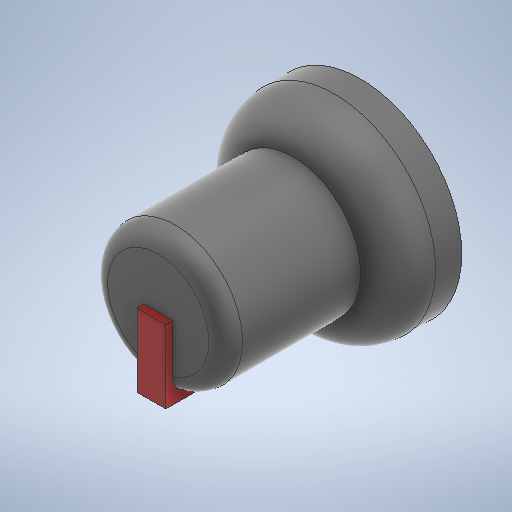
# Autodesk Inventor part: VOL KNOB
Saved by Autodesk Inventor 2025 (Build 290162000, 162)
## iProperties
Created: 2025-05-10
Part Number: VOL KNOB
Material: Generic
Document SubType Name: Modeling
Designer: thesn
Density: 1 g/cm^3
Appearance: Default
Author: thesn
Autodesk Inventor part; units mm, degrees
ref_plane "YZ Plane" through (0, 0, 0) normal (1, 0, 0) x (0, 1, 0)
ref_plane "XZ Plane" through (0, 0, 0) normal (0, 1, 0) x (-1, 0, 0)
ref_plane "XY Plane" through (0, 0, 0) normal (0, 0, 1) x (1, 0, 0)
sketch "Sketch1" plane through (0, 0, 0) normal (0, 0, 1) x (1, 0, 0)
  circle A0 centre (0, 0) radius 7.62
  circle A1 centre (0, 0) radius 5.08
  dimension "d0" = 15.24
  dimension "d1" = 10.16
  constraints: 2 centre point, 2 coincident
  measures "d0" diameter of A0
  measures "d1" diameter of A1
extrude "Extrusion1" add sketch "Sketch1" along normal blind 5.08 contours A0 | A1
extrude "Extrusion2" add sketch "Sketch1" along normal blind 15.24 contours A1
fillet "Fillet1" radius 3.175 1 edges at (-7.62, 0, 5.08)
fillet "Fillet2" radius 1.27 1 edges at (-5.08, 0, 15.24)
sketch "Sketch2" plane through (0, 0, 15.24) normal (0, 0, 1) x (1, 0, 0)
  line L0 (-1.0825, -0.0027) -> (1.0835, -0.0027)
  line L1 (1.0835, -0.0027) -> (1.0835, -5.4984)
  line L2 (1.0835, -5.4984) -> (-1.0825, -5.4984)
  line L3 (-1.0825, -5.4984) -> (-1.0825, -0.0027)
  point P0 (0, 0)
  point P1 (0.0005, -5.4984)
  point P2 (0.0005, -0.0027)
  dimension "d8" = 2.166
  dimension "d9" = 5.4958
  constraints: 8 end point, 2 midpoint, 2 parallel, 1 horizontal, 1 perpendicular
  measures "d8" distance between parallel lines of L1 L3
  measures "d9" distance of point (0, -5.498) point (0, -0.003)
extrude "Extrusion3" add sketch "Sketch2" along normal blind 0.508 and the other way blind 12.7
sketch "Sketch3" plane through (0, 0, 0) normal (0, 0, -1) x (-1, 0, 0)
  line L0 (-6.251, 1.1807) -> (3.3004, 1.1807) construction
  line L1 (3.3004, 1.1807) -> (3.3004, -0.1036) construction
  line L2 (3.3004, -0.1036) -> (-6.251, -0.1036) construction
  line L3 (-6.251, -0.1036) -> (-6.251, 1.1807) construction
  line L4 (-6.2543, 0.6467) -> (-6.083, 1.1547)
  line L5 (-6.083, 1.1547) -> (-5.9999, 1.1547)
  line L6 (-5.9999, 1.1547) -> (-5.8286, 0.6467)
  line L7 (-5.8286, 0.6467) -> (-5.8998, 0.6467)
  line L8 (-5.8998, 0.6467) -> (-5.9459, 0.7888)
  line L9 (-5.9459, 0.7888) -> (-6.1398, 0.7888)
  line L10 (-6.1398, 0.7888) -> (-6.1859, 0.6467)
  line L11 (-6.1859, 0.6467) -> (-6.2543, 0.6467)
  line L12 (-5.9645, 0.8464) -> (-6.0431, 1.0856)
  line L13 (-6.0431, 1.0856) -> (-6.1213, 0.8464)
  line L14 (-6.1213, 0.8464) -> (-5.9645, 0.8464)
  line L15 (-5.4923, 0.6467) -> (-5.5565, 0.6467)
  line L16 (-5.5565, 0.6467) -> (-5.5565, 0.6854)
  spline S0 degree 2 poles (-5.5565, 0.6854) (-5.5713, 0.6731) (-5.5931, 0.6566) (-5.608, 0.6496) knots 0 0 0 1 2 2 2
  spline S1 degree 2 poles (-5.608, 0.6496) (-5.6216, 0.643) (-5.6508, 0.636) (-5.6701, 0.636) knots 0 0 0 1 2 2 2
  spline S2 degree 2 poles (-5.6701, 0.636) (-5.7014, 0.636) (-5.7541, 0.662) (-5.7726, 0.6871) knots 0 0 0 1 2 2 2
  spline S3 degree 2 poles (-5.7726, 0.6871) (-5.7912, 0.7122) (-5.8117, 0.7863) (-5.8117, 0.8345) knots 0 0 0 1 2 2 2
  spline S4 degree 2 poles (-5.8117, 0.8345) (-5.8117, 0.8847) (-5.7858, 0.958) (-5.7632, 0.9855) knots 0 0 0 1 2 2 2
  spline S5 degree 2 poles (-5.7632, 0.9855) (-5.7422, 1.0102) (-5.6833, 1.0386) (-5.6508, 1.0386) knots 0 0 0 1 2 2 2
  spline S6 degree 2 poles (-5.6508, 1.0386) (-5.6224, 1.0386) (-5.58, 1.0259) (-5.5565, 1.0127) knots 0 0 0 1 2 2 2
  line L17 (-5.5565, 1.0127) -> (-5.5565, 1.1774)
  line L18 (-5.5565, 1.1774) -> (-5.4923, 1.1774)
  line L19 (-5.4923, 1.1774) -> (-5.4923, 0.6467)
  line L20 (-5.5565, 0.7394) -> (-5.5565, 0.9596)
  spline S7 degree 2 poles (-5.5565, 0.9596) (-5.5804, 0.9711) (-5.6183, 0.9798) (-5.6401, 0.9798) knots 0 0 0 1 2 2 2
  spline S8 degree 2 poles (-5.6401, 0.9798) (-5.6895, 0.9798) (-5.7455, 0.9057) (-5.7455, 0.8357) knots 0 0 0 1 2 2 2
  spline S9 degree 2 poles (-5.7455, 0.8357) (-5.7455, 0.7682) (-5.7026, 0.697) (-5.6553, 0.697) knots 0 0 0 1 2 2 2
  spline S10 degree 2 poles (-5.6553, 0.697) (-5.6302, 0.697) (-5.5791, 0.72) (-5.5565, 0.7394) knots 0 0 0 1 2 2 2
  spline S11 degree 2 poles (-5.1868, 0.6871) (-5.1946, 0.6813) (-5.221, 0.6607) (-5.2333, 0.6546) knots 0 0 0 1 2 2 2
  spline S12 degree 2 poles (-5.2333, 0.6546) (-5.2502, 0.6455) (-5.2819, 0.636) (-5.3107, 0.636) knots 0 0 0 1 2 2 2
  spline S13 degree 2 poles (-5.3107, 0.636) (-5.3342, 0.636) (-5.3766, 0.6537) (-5.3927, 0.6698) knots 0 0 0 1 2 2 2
  spline S14 degree 2 poles (-5.3927, 0.6698) (-5.4079, 0.6854) (-5.4264, 0.7315) (-5.4264, 0.7571) knots 0 0 0 1 2 2 2
  spline S15 degree 2 poles (-5.4264, 0.7571) (-5.4264, 0.7966) (-5.3931, 0.8526) (-5.3568, 0.8686) knots 0 0 0 1 2 2 2
  spline S16 degree 2 poles (-5.3568, 0.8686) (-5.3247, 0.8834) (-5.2375, 0.8946) (-5.1868, 0.8974) knots 0 0 0 1 2 2 2
  line L21 (-5.1868, 0.8974) -> (-5.1868, 0.9098)
  spline S17 degree 2 poles (-5.1868, 0.9098) (-5.1868, 0.932) (-5.2004, 0.9596) (-5.2128, 0.9674) knots 0 0 0 1 2 2 2
  spline S18 degree 2 poles (-5.2128, 0.9674) (-5.2251, 0.9752) (-5.2605, 0.9802) (-5.2795, 0.9802) knots 0 0 0 1 2 2 2
  spline S19 degree 2 poles (-5.2795, 0.9802) (-5.3017, 0.9802) (-5.3618, 0.967) (-5.3918, 0.9543) knots 0 0 0 1 2 2 2
  line L22 (-5.3918, 0.9543) -> (-5.3955, 0.9543)
  line L23 (-5.3955, 0.9543) -> (-5.3955, 1.0197)
  spline S20 degree 2 poles (-5.3955, 1.0197) (-5.3778, 1.0246) (-5.3116, 1.037) (-5.279, 1.037) knots 0 0 0 1 2 2 2
  spline S21 degree 2 poles (-5.279, 1.037) (-5.2395, 1.037) (-5.1856, 1.0246) (-5.1642, 1.0086) knots 0 0 0 1 2 2 2
  spline S22 degree 2 poles (-5.1642, 1.0086) (-5.1432, 0.9929) (-5.1226, 0.9431) (-5.1226, 0.9073) knots 0 0 0 1 2 2 2
  line L24 (-5.1226, 0.9073) -> (-5.1226, 0.6467)
  line L25 (-5.1226, 0.6467) -> (-5.1868, 0.6467)
  line L26 (-5.1868, 0.6467) -> (-5.1868, 0.6871)
  line L27 (-5.1868, 0.7406) -> (-5.1868, 0.8464)
  spline S23 degree 2 poles (-5.1868, 0.8464) (-5.2099, 0.8443) (-5.2795, 0.8373) (-5.3013, 0.8308) knots 0 0 0 1 2 2 2
  spline S24 degree 2 poles (-5.3013, 0.8308) (-5.3268, 0.8229) (-5.3601, 0.7904) (-5.3601, 0.7616) knots 0 0 0 1 2 2 2
  spline S25 degree 2 poles (-5.3601, 0.7616) (-5.3601, 0.7287) (-5.3231, 0.6953) (-5.2877, 0.6953) knots 0 0 0 1 2 2 2
  spline S26 degree 2 poles (-5.2877, 0.6953) (-5.2576, 0.6953) (-5.2082, 0.7212) (-5.1868, 0.7406) knots 0 0 0 1 2 2 2
  line L28 (-4.832, 1.1156) -> (-4.8353, 1.1156)
  spline S27 degree 2 poles (-4.8353, 1.1156) (-4.8439, 1.1189) (-4.876, 1.1247) (-4.8888, 1.1247) knots 0 0 0 1 2 2 2
  spline S28 degree 2 poles (-4.8888, 1.1247) (-4.9291, 1.1247) (-4.9637, 1.0885) (-4.9637, 1.0407) knots 0 0 0 1 2 2 2
  line L29 (-4.9637, 1.0407) -> (-4.9637, 1.0279)
  line L30 (-4.9637, 1.0279) -> (-4.8575, 1.0279)
  line L31 (-4.8575, 1.0279) -> (-4.8575, 0.9748)
  line L32 (-4.8575, 0.9748) -> (-4.9616, 0.9748)
  line L33 (-4.9616, 0.9748) -> (-4.9616, 0.6467)
  line L34 (-4.9616, 0.6467) -> (-5.0259, 0.6467)
  line L35 (-5.0259, 0.6467) -> (-5.0259, 0.9748)
  line L36 (-5.0259, 0.9748) -> (-5.0691, 0.9748)
  line L37 (-5.0691, 0.9748) -> (-5.0691, 1.0279)
  line L38 (-5.0691, 1.0279) -> (-5.0259, 1.0279)
  line L39 (-5.0259, 1.0279) -> (-5.0259, 1.0407)
  spline S29 degree 2 poles (-5.0259, 1.0407) (-5.0259, 1.109) (-4.9596, 1.1807) (-4.8978, 1.1807) knots 0 0 0 1 2 2 2
  spline S30 degree 2 poles (-4.8978, 1.1807) (-4.8801, 1.1807) (-4.846, 1.177) (-4.832, 1.1745) knots 0 0 0 1 2 2 2
  line L40 (-4.832, 1.1745) -> (-4.832, 1.1156)
  line L41 (-4.608, 0.9592) -> (-4.6113, 0.9592)
  spline S31 degree 2 poles (-4.6113, 0.9592) (-4.6187, 0.9613) (-4.6348, 0.9621) (-4.6459, 0.9621) knots 0 0 0 1 2 2 2
  spline S32 degree 2 poles (-4.6459, 0.9621) (-4.6718, 0.9621) (-4.7229, 0.9394) (-4.7459, 0.9172) knots 0 0 0 1 2 2 2
  line L42 (-4.7459, 0.9172) -> (-4.7459, 0.6467)
  line L43 (-4.7459, 0.6467) -> (-4.8102, 0.6467)
  line L44 (-4.8102, 0.6467) -> (-4.8102, 1.0279)
  line L45 (-4.8102, 1.0279) -> (-4.7459, 1.0279)
  line L46 (-4.7459, 1.0279) -> (-4.7459, 0.9711)
  spline S33 degree 2 poles (-4.7459, 0.9711) (-4.7109, 1.0024) (-4.6587, 1.0279) (-4.634, 1.0279) knots 0 0 0 1 2 2 2
  spline S34 degree 2 poles (-4.634, 1.0279) (-4.6241, 1.0279) (-4.6142, 1.0271) (-4.608, 1.0259) knots 0 0 0 1 2 2 2
  line L47 (-4.608, 1.0259) -> (-4.608, 0.9592)
  line L48 (-4.2618, 0.6467) -> (-4.326, 0.6467)
  line L49 (-4.326, 0.6467) -> (-4.326, 0.6887)
  spline S35 degree 2 poles (-4.326, 0.6887) (-4.3557, 0.6628) (-4.4088, 0.636) (-4.4417, 0.636) knots 0 0 0 1 2 2 2
  spline S36 degree 2 poles (-4.4417, 0.636) (-4.4664, 0.636) (-4.5105, 0.6525) (-4.5265, 0.6702) knots 0 0 0 1 2 2 2
  spline S37 degree 2 poles (-4.5265, 0.6702) (-4.543, 0.6879) (-4.5611, 0.7418) (-4.5611, 0.7805) knots 0 0 0 1 2 2 2
  line L50 (-4.5611, 0.7805) -> (-4.5611, 1.0279)
  line L51 (-4.5611, 1.0279) -> (-4.4969, 1.0279)
  line L52 (-4.4969, 1.0279) -> (-4.4969, 0.8106)
  spline S38 degree 2 poles (-4.4969, 0.8106) (-4.4969, 0.7801) (-4.4923, 0.7402) (-4.4845, 0.7254) knots 0 0 0 1 2 2 2
  spline S39 degree 2 poles (-4.4845, 0.7254) (-4.4767, 0.7105) (-4.4499, 0.697) (-4.4248, 0.697) knots 0 0 0 1 2 2 2
  spline S40 degree 2 poles (-4.4248, 0.697) (-4.4014, 0.697) (-4.3483, 0.7237) (-4.326, 0.7431) knots 0 0 0 1 2 2 2
  line L53 (-4.326, 0.7431) -> (-4.326, 1.0279)
  line L54 (-4.326, 1.0279) -> (-4.2618, 1.0279)
  line L55 (-4.2618, 1.0279) -> (-4.2618, 0.6467)
  line L56 (-4.1033, 0.6467) -> (-4.1675, 0.6467)
  line L57 (-4.1675, 0.6467) -> (-4.1675, 1.0279)
  line L58 (-4.1675, 1.0279) -> (-4.1033, 1.0279)
  line L59 (-4.1033, 1.0279) -> (-4.1033, 0.6467)
  line L60 (-4.0988, 1.0913) -> (-4.1717, 1.0913)
  line L61 (-4.1717, 1.0913) -> (-4.1717, 1.158)
  line L62 (-4.1717, 1.158) -> (-4.0988, 1.158)
  line L63 (-4.0988, 1.158) -> (-4.0988, 1.0913)
  spline S41 degree 2 poles (-3.8938, 0.6393) (-3.9461, 0.6393) (-4.0049, 0.699) (-4.0049, 0.7636) knots 0 0 0 1 2 2 2
  line L64 (-4.0049, 0.7636) -> (-4.0049, 0.9748)
  line L65 (-4.0049, 0.9748) -> (-4.0482, 0.9748)
  line L66 (-4.0482, 0.9748) -> (-4.0482, 1.0279)
  line L67 (-4.0482, 1.0279) -> (-4.0049, 1.0279)
  line L68 (-4.0049, 1.0279) -> (-4.0049, 1.1374)
  line L69 (-4.0049, 1.1374) -> (-3.9407, 1.1374)
  line L70 (-3.9407, 1.1374) -> (-3.9407, 1.0279)
  line L71 (-3.9407, 1.0279) -> (-3.8226, 1.0279)
  line L72 (-3.8226, 1.0279) -> (-3.8226, 0.9748)
  line L73 (-3.8226, 0.9748) -> (-3.9407, 0.9748)
  line L74 (-3.9407, 0.9748) -> (-3.9407, 0.7933)
  spline S42 degree 2 poles (-3.9407, 0.7933) (-3.9407, 0.7645) (-3.9386, 0.7328) (-3.9316, 0.7192) knots 0 0 0 1 2 2 2
  spline S43 degree 2 poles (-3.9316, 0.7192) (-3.9259, 0.7073) (-3.8999, 0.6953) (-3.8777, 0.6953) knots 0 0 0 1 2 2 2
  spline S44 degree 2 poles (-3.8777, 0.6953) (-3.8621, 0.6953) (-3.8328, 0.7048) (-3.8263, 0.7077) knots 0 0 0 1 2 2 2
  line L75 (-3.8263, 0.7077) -> (-3.8226, 0.7077)
  line L76 (-3.8226, 0.7077) -> (-3.8226, 0.65)
  spline S45 degree 2 poles (-3.8226, 0.65) (-3.8407, 0.6451) (-3.8777, 0.6393) (-3.8938, 0.6393) knots 0 0 0 1 2 2 2
  spline S46 degree 2 poles (-3.231, 1.0016) (-3.231, 0.9687) (-3.2545, 0.9094) (-3.2754, 0.8888) knots 0 0 0 1 2 2 2
  spline S47 degree 2 poles (-3.2754, 0.8888) (-3.3018, 0.8629) (-3.373, 0.8361) (-3.4274, 0.8361) knots 0 0 0 1 2 2 2
  line L77 (-3.4274, 0.8361) -> (-3.4846, 0.8361)
  line L78 (-3.4846, 0.8361) -> (-3.4846, 0.6467)
  line L79 (-3.4846, 0.6467) -> (-3.5521, 0.6467)
  line L80 (-3.5521, 0.6467) -> (-3.5521, 1.1547)
  line L81 (-3.5521, 1.1547) -> (-3.4245, 1.1547)
  spline S48 degree 2 poles (-3.4245, 1.1547) (-3.3792, 1.1547) (-3.3158, 1.1399) (-3.2915, 1.123) knots 0 0 0 1 2 2 2
  spline S49 degree 2 poles (-3.2915, 1.123) (-3.2631, 1.1037) (-3.231, 1.044) (-3.231, 1.0016) knots 0 0 0 1 2 2 2
  spline S50 degree 2 poles (-3.3014, 0.9995) (-3.3014, 1.0259) (-3.3195, 1.0646) (-3.338, 1.0769) knots 0 0 0 1 2 2 2
  spline S51 degree 2 poles (-3.338, 1.0769) (-3.3541, 1.0876) (-3.3969, 1.0963) (-3.4286, 1.0963) knots 0 0 0 1 2 2 2
  line L82 (-3.4286, 1.0963) -> (-3.4846, 1.0963)
  line L83 (-3.4846, 1.0963) -> (-3.4846, 0.8937)
  line L84 (-3.4846, 0.8937) -> (-3.4385, 0.8937)
  spline S52 degree 2 poles (-3.4385, 0.8937) (-3.3973, 0.8937) (-3.3467, 0.9069) (-3.3302, 0.9242) knots 0 0 0 1 2 2 2
  spline S53 degree 2 poles (-3.3302, 0.9242) (-3.315, 0.9394) (-3.3014, 0.9752) (-3.3014, 0.9995) knots 0 0 0 1 2 2 2
  line L85 (-2.9897, 0.6467) -> (-3.1865, 0.6467)
  line L86 (-3.1865, 0.6467) -> (-3.1865, 0.6986)
  line L87 (-3.1865, 0.6986) -> (-3.1219, 0.6986)
  line L88 (-3.1219, 0.6986) -> (-3.1219, 1.1029)
  line L89 (-3.1219, 1.1029) -> (-3.1865, 1.1029)
  line L90 (-3.1865, 1.1029) -> (-3.1865, 1.1547)
  line L91 (-3.1865, 1.1547) -> (-2.9897, 1.1547)
  line L92 (-2.9897, 1.1547) -> (-2.9897, 1.1029)
  line L93 (-2.9897, 1.1029) -> (-3.0544, 1.1029)
  line L94 (-3.0544, 1.1029) -> (-3.0544, 0.6986)
  line L95 (-3.0544, 0.6986) -> (-2.9897, 0.6986)
  line L96 (-2.9897, 0.6986) -> (-2.9897, 0.6467)
  spline S54 degree 2 poles (-2.5056, 0.9003) (-2.5056, 0.8308) (-2.562, 0.7188) (-2.6094, 0.6875) knots 0 0 0 1 2 2 2
  spline S55 degree 2 poles (-2.6094, 0.6875) (-2.6481, 0.6632) (-2.7275, 0.6467) (-2.7893, 0.6467) knots 0 0 0 1 2 2 2
  line L97 (-2.7893, 0.6467) -> (-2.9062, 0.6467)
  line L98 (-2.9062, 0.6467) -> (-2.9062, 1.1547)
  line L99 (-2.9062, 1.1547) -> (-2.7905, 1.1547)
  spline S56 degree 2 poles (-2.7905, 1.1547) (-2.7189, 1.1547) (-2.6374, 1.1333) (-2.6085, 1.1144) knots 0 0 0 1 2 2 2
  spline S57 degree 2 poles (-2.6085, 1.1144) (-2.5596, 1.0819) (-2.5056, 0.9744) (-2.5056, 0.9003) knots 0 0 0 1 2 2 2
  spline S58 degree 2 poles (-2.576, 0.9011) (-2.576, 0.9596) (-2.6147, 1.0423) (-2.653, 1.0658) knots 0 0 0 1 2 2 2
  spline S59 degree 2 poles (-2.653, 1.0658) (-2.6802, 1.0819) (-2.7415, 1.0963) (-2.7872, 1.0963) knots 0 0 0 1 2 2 2
  line L100 (-2.7872, 1.0963) -> (-2.8387, 1.0963)
  line L101 (-2.8387, 1.0963) -> (-2.8387, 0.7052)
  line L102 (-2.8387, 0.7052) -> (-2.7872, 0.7052)
  spline S60 degree 2 poles (-2.7872, 0.7052) (-2.7423, 0.7052) (-2.6744, 0.7196) (-2.6468, 0.7389) knots 0 0 0 1 2 2 2
  spline S61 degree 2 poles (-2.6468, 0.7389) (-2.6114, 0.7628) (-2.576, 0.8419) (-2.576, 0.9011) knots 0 0 0 1 2 2 2
  line L103 (-2.3196, 0.6467) -> (-2.4011, 0.6467)
  line L104 (-2.4011, 0.6467) -> (-2.4011, 0.7439)
  line L105 (-2.4011, 0.7439) -> (-2.3196, 0.7439)
  line L106 (-2.3196, 0.7439) -> (-2.3196, 0.6467)
  line L107 (-2.3196, 0.9308) -> (-2.4011, 0.9308)
  line L108 (-2.4011, 0.9308) -> (-2.4011, 1.0279)
  line L109 (-2.4011, 1.0279) -> (-2.3196, 1.0279)
  line L110 (-2.3196, 1.0279) -> (-2.3196, 0.9308)
  line L111 (-1.6683, 0.6467) -> (-1.9816, 0.6467)
  line L112 (-1.9816, 0.6467) -> (-1.9816, 0.7188)
  spline S62 degree 2 poles (-1.9816, 0.7188) (-1.9478, 0.7505) (-1.8877, 0.8093) (-1.8589, 0.841) knots 0 0 0 1 2 2 2
  spline S63 degree 2 poles (-1.8589, 0.841) (-1.8008, 0.9049) (-1.7584, 0.9814) (-1.7584, 1.0222) knots 0 0 0 1 2 2 2
  spline S64 degree 2 poles (-1.7584, 1.0222) (-1.7584, 1.0436) (-1.7716, 1.0757) (-1.7836, 1.086) knots 0 0 0 1 2 2 2
  spline S65 degree 2 poles (-1.7836, 1.086) (-1.7955, 1.0963) (-1.8268, 1.1066) (-1.8457, 1.1066) knots 0 0 0 1 2 2 2
  spline S66 degree 2 poles (-1.8457, 1.1066) (-1.8638, 1.1066) (-1.9009, 1.0975) (-1.9178, 1.0905) knots 0 0 0 1 2 2 2
  spline S67 degree 2 poles (-1.9178, 1.0905) (-1.9322, 1.0848) (-1.9589, 1.0683) (-1.9672, 1.0625) knots 0 0 0 1 2 2 2
  line L113 (-1.9672, 1.0625) -> (-1.9709, 1.0625)
  line L114 (-1.9709, 1.0625) -> (-1.9709, 1.135)
  spline S68 degree 2 poles (-1.9709, 1.135) (-1.9499, 1.1453) (-1.8745, 1.1654) (-1.8408, 1.1654) knots 0 0 0 1 2 2 2
  spline S69 degree 2 poles (-1.8408, 1.1654) (-1.7696, 1.1654) (-1.6893, 1.0901) (-1.6893, 1.0259) knots 0 0 0 1 2 2 2
  spline S70 degree 2 poles (-1.6893, 1.0259) (-1.6893, 0.9958) (-1.7033, 0.9456) (-1.7156, 0.9242) knots 0 0 0 1 2 2 2
  spline S71 degree 2 poles (-1.7156, 0.9242) (-1.728, 0.902) (-1.7638, 0.8583) (-1.7836, 0.8373) knots 0 0 0 1 2 2 2
  spline S72 degree 2 poles (-1.7836, 0.8373) (-1.8157, 0.8023) (-1.8943, 0.7274) (-1.9178, 0.7056) knots 0 0 0 1 2 2 2
  line L115 (-1.9178, 0.7056) -> (-1.6683, 0.7056)
  line L116 (-1.6683, 0.7056) -> (-1.6683, 0.6467)
  spline S73 degree 2 poles (-1.2842, 0.9007) (-1.2842, 0.7641) (-1.3637, 0.636) (-1.4464, 0.636) knots 0 0 0 1 2 2 2
  spline S74 degree 2 poles (-1.4464, 0.636) (-1.5304, 0.636) (-1.609, 0.7665) (-1.609, 0.9003) knots 0 0 0 1 2 2 2
  spline S75 degree 2 poles (-1.609, 0.9003) (-1.609, 1.0378) (-1.5296, 1.165) (-1.4464, 1.165) knots 0 0 0 1 2 2 2
  spline S76 degree 2 poles (-1.4464, 1.165) (-1.3628, 1.165) (-1.2842, 1.0333) (-1.2842, 0.9007) knots 0 0 0 1 2 2 2
  spline S77 degree 2 poles (-1.3715, 0.7459) (-1.3616, 0.7711) (-1.3534, 0.8485) (-1.3534, 0.9007) knots 0 0 0 1 2 2 2
  spline S78 degree 2 poles (-1.3534, 0.9007) (-1.3534, 0.953) (-1.3616, 1.03) (-1.3719, 1.0559) knots 0 0 0 1 2 2 2
  spline S79 degree 2 poles (-1.3719, 1.0559) (-1.3822, 1.0819) (-1.418, 1.1086) (-1.4464, 1.1086) knots 0 0 0 1 2 2 2
  spline S80 degree 2 poles (-1.4464, 1.1086) (-1.4748, 1.1086) (-1.5114, 1.0819) (-1.5221, 1.0551) knots 0 0 0 1 2 2 2
  spline S81 degree 2 poles (-1.5221, 1.0551) (-1.5324, 1.0292) (-1.5398, 0.9501) (-1.5398, 0.9003) knots 0 0 0 1 2 2 2
  spline S82 degree 2 poles (-1.5398, 0.9003) (-1.5398, 0.8468) (-1.5333, 0.7752) (-1.5226, 0.7472) knots 0 0 0 1 2 2 2
  spline S83 degree 2 poles (-1.5226, 0.7472) (-1.5127, 0.7208) (-1.476, 0.6924) (-1.4464, 0.6924) knots 0 0 0 1 2 2 2
  spline S84 degree 2 poles (-1.4464, 0.6924) (-1.4184, 0.6924) (-1.3818, 0.7192) (-1.3715, 0.7459) knots 0 0 0 1 2 2 2
  line L117 (-0.8923, 0.8213) -> (-0.9528, 0.8213)
  line L118 (-0.9528, 0.8213) -> (-0.9528, 0.6467)
  line L119 (-0.9528, 0.6467) -> (-1.0183, 0.6467)
  line L120 (-1.0183, 0.6467) -> (-1.0183, 0.8213)
  line L121 (-1.0183, 0.8213) -> (-1.2426, 0.8213)
  line L122 (-1.2426, 0.8213) -> (-1.2426, 0.8929)
  line L123 (-1.2426, 0.8929) -> (-1.0154, 1.1547)
  line L124 (-1.0154, 1.1547) -> (-0.9528, 1.1547)
  line L125 (-0.9528, 1.1547) -> (-0.9528, 0.876)
  line L126 (-0.9528, 0.876) -> (-0.8923, 0.876)
  line L127 (-0.8923, 0.876) -> (-0.8923, 0.8213)
  line L128 (-1.0183, 0.876) -> (-1.0183, 1.0745)
  line L129 (-1.0183, 1.0745) -> (-1.1891, 0.876)
  line L130 (-1.1891, 0.876) -> (-1.0183, 0.876)
  spline S85 degree 2 poles (-0.5169, 0.8114) (-0.5169, 0.7723) (-0.5428, 0.706) (-0.5646, 0.6838) knots 0 0 0 1 2 2 2
  spline S86 degree 2 poles (-0.5646, 0.6838) (-0.5872, 0.6603) (-0.6441, 0.636) (-0.6782, 0.636) knots 0 0 0 1 2 2 2
  spline S87 degree 2 poles (-0.6782, 0.636) (-0.7124, 0.636) (-0.7688, 0.6591) (-0.7902, 0.6821) knots 0 0 0 1 2 2 2
  spline S88 degree 2 poles (-0.7902, 0.6821) (-0.8165, 0.7097) (-0.8462, 0.8023) (-0.8462, 0.8699) knots 0 0 0 1 2 2 2
  spline S89 degree 2 poles (-0.8462, 0.8699) (-0.8462, 0.9361) (-0.819, 1.0428) (-0.7906, 1.0823) knots 0 0 0 1 2 2 2
  spline S90 degree 2 poles (-0.7906, 1.0823) (-0.763, 1.121) (-0.6758, 1.1642) (-0.6185, 1.1642) knots 0 0 0 1 2 2 2
  spline S91 degree 2 poles (-0.6185, 1.1642) (-0.6017, 1.1642) (-0.572, 1.1609) (-0.5609, 1.1572) knots 0 0 0 1 2 2 2
  line L131 (-0.5609, 1.1572) -> (-0.5609, 1.0918)
  line L132 (-0.5609, 1.0918) -> (-0.5638, 1.0918)
  spline S92 degree 2 poles (-0.5638, 1.0918) (-0.5732, 1.0967) (-0.6078, 1.1053) (-0.6276, 1.1053) knots 0 0 0 1 2 2 2
  spline S93 degree 2 poles (-0.6276, 1.1053) (-0.691, 1.1053) (-0.7688, 1.0197) (-0.7762, 0.9357) knots 0 0 0 1 2 2 2
  spline S94 degree 2 poles (-0.7762, 0.9357) (-0.7519, 0.9526) (-0.7009, 0.9711) (-0.6704, 0.9711) knots 0 0 0 1 2 2 2
  spline S95 degree 2 poles (-0.6704, 0.9711) (-0.6408, 0.9711) (-0.5963, 0.9592) (-0.572, 0.9411) knots 0 0 0 1 2 2 2
  spline S96 degree 2 poles (-0.572, 0.9411) (-0.544, 0.9201) (-0.5169, 0.855) (-0.5169, 0.8114) knots 0 0 0 1 2 2 2
  spline S97 degree 2 poles (-0.586, 0.8085) (-0.586, 0.8398) (-0.6025, 0.8822) (-0.6206, 0.897) knots 0 0 0 1 2 2 2
  spline S98 degree 2 poles (-0.6206, 0.897) (-0.6342, 0.9077) (-0.6679, 0.9147) (-0.6856, 0.9147) knots 0 0 0 1 2 2 2
  spline S99 degree 2 poles (-0.6856, 0.9147) (-0.7095, 0.9147) (-0.7544, 0.9003) (-0.7762, 0.8867) knots 0 0 0 1 2 2 2
  spline S100 degree 2 poles (-0.7762, 0.8867) (-0.7766, 0.8793) (-0.7774, 0.8653) (-0.7774, 0.8546) knots 0 0 0 1 2 2 2
  spline S101 degree 2 poles (-0.7774, 0.8546) (-0.7774, 0.8019) (-0.7569, 0.7373) (-0.7412, 0.7204) knots 0 0 0 1 2 2 2
  spline S102 degree 2 poles (-0.7412, 0.7204) (-0.7268, 0.7044) (-0.6955, 0.6916) (-0.6778, 0.6916) knots 0 0 0 1 2 2 2
  spline S103 degree 2 poles (-0.6778, 0.6916) (-0.6366, 0.6916) (-0.586, 0.7501) (-0.586, 0.8085) knots 0 0 0 1 2 2 2
  point P0 (0, 0)
  constraints: 2 other
extrude "Extrusion4" cut sketch "Sketch3" against normal blind 0.508
body "Solid1"
